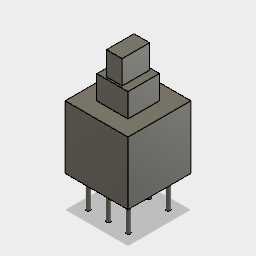
Button_Push v1 (Autodesk Fusion 360 design; units mm, degrees)
Autodesk Fusion 360 part; units mm, degrees
sketch "Sketch1" plane through (0, 0, 0) normal (0, 1, 0) x (1, 0, 0)
  line L0 (0, 0) -> (-8, 0)
  line L1 (-8, 0) -> (-8, 8)
  line L2 (-8, 8) -> (0, 8)
  line L3 (0, 8) -> (0, 0)
  line L4 (-4.9967, 2.2502) -> (-3, 2.2502)
  line L5 (-3, 2.2502) -> (-3, 5.7645)
  line L6 (-3, 5.7645) -> (-4.9967, 5.7645)
  line L7 (-4.9967, 5.7645) -> (-4.9967, 2.2502)
  line L8 (-5.9662, 2) -> (-2, 2)
  line L9 (-2, 2) -> (-2, 6.0099)
  line L10 (-2, 6.0099) -> (-5.9662, 6.0099)
  line L11 (-5.9662, 6.0099) -> (-5.9662, 2)
  circle A0 centre (-4, 1.5) radius 0.27
  circle A1 centre (-1.46, 1.5) radius 0.27
  circle A2 centre (-6.54, 1.5) radius 0.27
  circle A3 centre (-6.54, 6.58) radius 0.27
  circle A4 centre (-4, 6.58) radius 0.27
  circle A5 centre (-1.46, 6.58) radius 0.27
  dimension "d1" = 8
  dimension "d2" = 8
  constraint horizontal L0
  constraint vertical L1
  constraint horizontal L2
  constraint vertical L3
  constraint horizontal L4
  constraint vertical L5
  constraint horizontal L6
  constraint vertical L7
  constraint horizontal L8
  constraint vertical L9
  constraint horizontal L10
  constraint vertical L11
extrude "Extrude1" add sketch "Sketch1" along normal blind 8 contours L0 L1 L2 L3 | A0 | A1 | A2 | A3 | A4 | A5
extrude "Extrude2" add sketch "Sketch1" along normal blind 11 contours L8 L9 L10 L11
extrude "Extrude3" add sketch "Sketch1" along normal blind 14 contours L4 L5 L6 L7
move_body "MoveBody1" bodies 1 to x (1, 0, 0) y (0, 1, 0) z (0, 0, 1) at (0, 4, 0)
extrude "Extrude4" add sketch "Sketch1" along normal blind 4 contours A0 | A1 | A2 | A3 | A4 | A5
